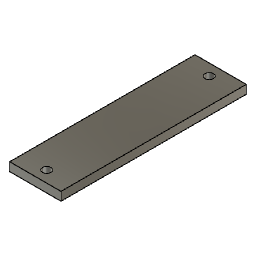
TopFlap v2 (Autodesk Fusion 360 design; units mm, degrees)
Autodesk Fusion 360 part; units mm, degrees
sketch "Sketch1" plane through (0, 0, 0) normal (0, 0, 1) x (1, 0, 0)
  line L0 (0, 0) -> (18, 0)
  line L1 (18, 0) -> (18, 65)
  line L2 (18, 65) -> (0, 65)
  line L3 (0, 65) -> (0, 0)
  circle A0 centre (9, 4) radius 1.5
  circle A1 centre (9, 61) radius 1.5
  dimension "d1" = 18
  dimension "d2" = 65
  dimension "d4" = 3
  dimension "d5" = 4
  dimension "d6" = 9
  dimension "d7" = 3
  dimension "d8" = 4
  dimension "d9" = 9
  constraint horizontal L0
  constraint vertical L1
  constraint horizontal L2
  constraint vertical L3
  constraint coincident L0.start L3.end
  measures "d1" distance of L0.start L0.end
  measures "d2" distance of L0.start L2.end
  measures "d4" diameter of A0
  measures "d5" distance of L0 A0.centre
  measures "d6" distance of L1 A0.centre
  measures "d7" diameter of A1
  measures "d8" distance of L2 A1.centre
  measures "d9" distance of L1 A1.centre
extrude "Extrude1" add sketch "Sketch1" along normal blind 3
equation "ScrewHole = 3 mm"
equation "d4 = ScrewHole"
equation "d7 = ScrewHole"
